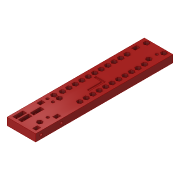
# Autodesk Inventor part: Coupler lift long for bracket right
Saved by Autodesk Inventor 2020 (Build 240168000, 168)
## iProperties
Created: 2019-10-02
Part Number: Coupler lift long for bracket right
Material: Generic
Document SubType Name: Modeling
Designer: ball
Density: 1 g/cm^3
Appearance: Default
Author: ball
Autodesk Inventor part; units mm, degrees
ref_plane "YZ Plane" through (0, 0, 0) normal (1, 0, 0) x (0, 1, 0)
ref_plane "XZ Plane" through (0, 0, 0) normal (0, 1, 0) x (-1, 0, 0)
ref_plane "XY Plane" through (0, 0, 0) normal (0, 0, 1) x (1, 0, 0)
sketch "Sketch1" plane through (0, 0, 0) normal (0, 1, 0) x (-1, 0, 0)
  line L0 (0, 0) -> (35.5, 0)
  line L1 (35.5, 0) -> (35.5, -170)
  line L2 (35.5, -170) -> (0, -170)
  line L3 (0, -170) -> (0, 0)
  dimension "d0" = 35.5
  dimension "d1" = 170
  constraints: 8 end point, 2 parallel, 1 horizontal, 1 perpendicular
  measures "d0" distance of L1.end L2.end
  measures "d1" distance of L0.end L1.end
extrude "BlockShape" add sketch "Sketch1" along normal blind 9
sketch "Sketch2" plane through (0, 9, 0) normal (0, 1, 0) x (1, 0, 0)
  circle A0 centre (-10, 15) radius 3.25 construction
  line L0 (-35.5, 0) -> (0, 0) projected
  line L1 (0, 0) -> (0, 170) projected
  line L2 (-13.25, 15) -> (-11.625, 17.8146)
  line L3 (-11.625, 17.8146) -> (-8.375, 17.8146)
  line L4 (-8.375, 17.8146) -> (-6.75, 15)
  line L5 (-6.75, 15) -> (-8.375, 12.1854)
  line L6 (-8.375, 12.1854) -> (-11.625, 12.1854)
  line L7 (-11.625, 12.1854) -> (-13.25, 15)
  circle A1 centre (-10, 150) radius 3.25 construction
  line L8 (-13.25, 150) -> (-11.625, 152.8146)
  line L9 (-11.625, 152.8146) -> (-8.375, 152.8146)
  line L10 (-8.375, 152.8146) -> (-6.75, 150)
  line L11 (-6.75, 150) -> (-8.375, 147.1854)
  line L12 (-8.375, 147.1854) -> (-11.625, 147.1854)
  line L13 (-11.625, 147.1854) -> (-13.25, 150)
  line L14 (0, 170) -> (-35.5, 170) projected
  circle A2 centre (-10, 15) radius 1.7 construction
  circle A3 centre (-10, 150) radius 1.7 construction
  dimension "d7" = 6.5
  dimension "d10" = 6.5
  dimension "d23" = 135
  dimension "d24" = 15
  dimension "d25" = 10
  dimension "d28" = 3.4
  dimension "d29" = 3.4
  constraints: 24 end point, 4 coincident, 2 centre point, 2 horizontal alignment, 30 other
  measures "d23" distance of point (-10, 150) point (-10, 15)
  measures "d24" distance from line of L0 point (-10, 15)
  measures "d25" distance from line of L1 point (-10, 15)
  measures "d28" diameter of A2
  measures "d29" diameter of A3
extrude "SlideNutWell2" cut sketch "Sketch2" against normal blind 5
sketch "Sketch3" plane through (0, 0, 0) normal (0, -1, 0) x (1, 0, 0)
  circle A0 centre (-10, -25) radius 3.25 construction
  line L0 (0, 0) -> (-35.5, 0) projected
  line L1 (-35.5, 0) -> (-35.5, -170) projected
  line L2 (-11.6286, -27.8125) -> (-13.25, -24.9958)
  line L3 (-13.25, -24.9958) -> (-11.6214, -22.1833)
  line L4 (-11.6214, -22.1833) -> (-8.3714, -22.1875)
  line L5 (-8.3714, -22.1875) -> (-6.75, -25.0042)
  line L6 (-6.75, -25.0042) -> (-8.3786, -27.8167)
  line L7 (-8.3786, -27.8167) -> (-11.6286, -27.8125)
  circle A1 centre (-10, -160) radius 3.25 construction
  line L8 (-6.75, -160) -> (-8.375, -162.8146)
  line L9 (-8.375, -162.8146) -> (-11.625, -162.8146)
  line L10 (-11.625, -162.8146) -> (-13.25, -160)
  line L11 (-13.25, -160) -> (-11.625, -157.1854)
  line L12 (-11.625, -157.1854) -> (-8.375, -157.1854)
  line L13 (-8.375, -157.1854) -> (-6.75, -160)
  line L14 (0, -170) -> (0, 0) projected
  dimension "d15" = 6.5
  dimension "d18" = 6.5
  dimension "d16" = 25
  dimension "d19" = 135
  dimension "d26" = 10
  dimension "d27" = 10
  constraints: 24 end point, 2 coincident, 1 horizontal alignment, 31 other
  measures "d16" distance from line of L0 point (-10, -25)
  measures "d19" distance of point (-10, -160) point (-10, -25)
  measures "d26" distance from line of L14 point (-10, -25)
  measures "d27" distance from line of L14 point (-10, -160)
extrude "SlideNutWell1" cut sketch "Sketch3" against normal blind 5
sketch "Sketch5" plane through (0, 9, 0) normal (0, 1, 0) x (1, 0, 0)
  circle A0 centre (-10, 15) radius 1.7
  line L0 (0, 0) -> (0, 170) projected
  line L1 (-35.5, 0) -> (0, 0) projected
  circle A1 centre (-10, 150) radius 1.7
  circle A2 centre (-10, 25) radius 1.7
  circle A3 centre (-10, 160) radius 1.7
  dimension "d30" = 3.4
  dimension "d31" = 10
  dimension "d32" = 15
  dimension "d33" = 3.4
  dimension "d34" = 10
  dimension "d35" = 135
  dimension "d36" = 3.4
  dimension "d37" = 25
  dimension "d38" = 3.4
  dimension "d39" = 10
  dimension "d40" = 135
  constraints: 4 centre point
  measures "d30" diameter of A0
  measures "d31" distance from line of L0 A0.centre
  measures "d32" distance from line of L1 A0.centre
  measures "d33" diameter of A1
  measures "d34" distance from line of L0 A1.centre
  measures "d35" distance of A1.centre A0.centre
  measures "d36" diameter of A2
  measures "d37" distance from line of L1 A2.centre
  measures "d38" diameter of A3
  measures "d39" distance from line of L0 A3.centre
  measures "d40" distance of A2.centre A3.centre
extrude "SlideMoutingHoles" cut sketch "Sketch5" against normal through all
sketch "Sketch6" plane through (0, 9, 0) normal (0, 1, 0) x (1, 0, 0)
  line L0 (-32.5, 4) -> (-27.7502, 4)
  line L1 (-27.7502, 4) -> (-27.7502, 16.7)
  line L2 (-27.7502, 16.7) -> (-32.5, 16.7)
  line L3 (-32.5, 16.7) -> (-32.5, 4)
  line L4 (-35.5, 0) -> (0, 0) projected
  line L5 (-35.5, 170) -> (-35.5, 0) projected
  line L6 (-25.7502, 4) -> (-21.0002, 4)
  line L7 (-21.0002, 4) -> (-21.0002, 16.7)
  line L8 (-21.0002, 16.7) -> (-25.7502, 16.7)
  line L9 (-25.7502, 16.7) -> (-25.7502, 4)
  line L10 (0, 0) -> (0, 170) construction
  line L11 (-35.5, 170) -> (0, 170) projected
  line L12 (0, 0) -> (-20, 0) construction
  line L13 (-20, 0) -> (-20, 170) construction
  line L14 (-20, 170) -> (0, 170) construction
  line L15 (0, 170) -> (0, 0)
  circle A0 centre (-23.3752, 44.7) radius 1.7
  circle A1 centre (-30.125, 44.7) radius 1.7
  circle A2 centre (-30.125, 52.7) radius 1.7
  circle A3 centre (-23.3752, 52.7) radius 1.7
  line L16 (-25.7502, 18.7) -> (-21.0002, 18.7)
  line L17 (-21.0002, 18.7) -> (-21.0002, 31.4)
  line L18 (-21.0002, 31.4) -> (-25.7502, 31.4)
  line L19 (-25.7502, 31.4) -> (-25.7502, 18.7)
  dimension "d43" = 4.7498
  dimension "d44" = 12.7
  dimension "d45" = 4
  dimension "d46" = 3
  dimension "d47" = 4.75
  dimension "d48" = 2
  dimension "d49" = 20
  dimension "d50" = 3.4
  dimension "d51" = 28
  dimension "d87" = 3.4
  dimension "d88" = 5.375
  dimension "d90" = 3.4
  dimension "d91" = 8
  dimension "d92" = 3.4
  dimension "d180" = 4.75
  dimension "d181" = 12.7
  dimension "d182" = 2
  dimension "d183" = 12.7
  dimension "d184" = 4
  dimension "d260" = 28
  dimension "d261" = 8
  constraints: 32 end point, 8 parallel, 4 centre point, 4 horizontal, 4 perpendicular, 2 point on line
  measures "d43" distance of L2.end L1.end
  measures "d44" distance of L1.end L0.end
  measures "d45" distance between parallel lines of L4 L0
  measures "d46" distance between parallel lines of L5 L3
  measures "d47" distance of L8.end L7.end
  measures "d48" distance between parallel lines of L9 L1
  measures "d49" distance of L13.end L14.end
  measures "d50" diameter of A0
  measures "d51" distance from line of A0.centre L8
  measures "d87" diameter of A1
  measures "d88" distance from line of L5 A1.centre
  measures "d90" diameter of A2
  measures "d91" distance of A2.centre A1.centre
  measures "d92" diameter of A3
  measures "d180" distance of L18.end L17.end
  measures "d181" distance of L17.end L16.end
  measures "d182" distance between parallel lines of L16 L8
  measures "d183" distance between parallel lines of L8 L6
  measures "d184" distance between parallel lines of L4 L6
  measures "d260" distance from line of L2 A1.centre
  measures "d261" distance of A0.centre A3.centre
extrude "PulleyHoles" cut sketch "Sketch6" against normal through all contours L3 L2 L1 L0 | L9 L8 L7 L6 | A0 | A1 | A2 | A3 | L19 L18 L17 L16
sketch "Sketch7" plane through (0, 0, 0) normal (0, -1, 0) x (1, 0, 0)
  circle A0 centre (-23.3752, -44.7) radius 1.7 projected
  circle A1 centre (-23.3752, -44.7) radius 3.25 construction
  circle A2 centre (-30.1625, -44.7) radius 3.25 construction
  line L0 (-30.125, -41.4502) -> (-27.3294, -43.1076)
  line L1 (-27.3294, -43.1076) -> (-27.3669, -46.3574)
  line L2 (-27.3669, -46.3574) -> (-30.2, -47.9498)
  line L3 (-30.2, -47.9498) -> (-32.9956, -46.2924)
  line L4 (-32.9956, -46.2924) -> (-32.9581, -43.0426)
  line L5 (-32.9581, -43.0426) -> (-30.125, -41.4502)
  circle A3 centre (-30.125, -44.7) radius 1.7 projected
  line L6 (-20.1252, -44.7) -> (-21.7502, -47.5146)
  line L7 (-21.7502, -47.5146) -> (-25.0002, -47.5146)
  line L8 (-25.0002, -47.5146) -> (-26.6252, -44.7)
  line L9 (-26.6252, -44.7) -> (-25.0002, -41.8854)
  line L10 (-25.0002, -41.8854) -> (-21.7502, -41.8854)
  line L11 (-21.7502, -41.8854) -> (-20.1252, -44.7)
  point P0 (0, 0)
  dimension "d54" = 6.5
  dimension "d89" = 6.5
  dimension "d262" = 0
  constraints: 24 end point, 4 coincident, 1 horizontal alignment, 32 other
  measures "d262" vertical distance of point (-30.162, -44.7) A3.centre
extrude "TensionNutWells2" cut sketch "Sketch7" against normal blind 5 contours A0 | L0 L1 L2 L3 L4 L5 | A3 | L6 L7 L8 L9 L10 L11
sketch "Sketch8" plane through (-35.5, 0, -170) normal (-1, 0, 0) x (0, 0, 1)
  circle A0 centre (159.65, 4.5) radius 1.4605
  line L0 (0, 9) -> (170, 9) projected
  line L1 (170, 0) -> (170, 9) projected
  circle A1 centre (144.95, 4.5) radius 1.45
  dimension "d57" = 2.921
  dimension "d58" = 4.5
  dimension "d59" = 10.35
  dimension "d185" = 2.9
  dimension "d186" = 14.7
  dimension "d187" = 4.5
  constraints: 2 centre point
  measures "d57" diameter of A0
  measures "d58" distance from line of L0 A0.centre
  measures "d59" distance from line of L1 A0.centre
  measures "d185" diameter of A1
  measures "d186" distance of A1.centre A0.centre
  measures "d187" distance from line of L0 A1.centre
hole "PulleyMountingHole" at (-35.5, 4.5, -10.35) at (-35.5, 4.5, -25.05) direction (1, 0, 0) diameter 2.921 depth 21 counterbore diameter 3.4 counterbore depth 1.5
sketch "Sketch9" plane through (-21.0002, 9, -16.7) normal (-1, 0, 0) x (0, 0, 1)
  circle A0 centre (6.35, -4.5) radius 1.4605 projected
  circle A1 centre (6.35, -4.5) radius 2.54
  circle A2 centre (-8.35, -4.5) radius 1.4605 projected
  circle A3 centre (-8.35, -4.5) radius 2.54
  point P0 (16.7, -9)
  dimension "d67" = 5.08
  dimension "d194" = 5.08
  constraints: 2 centre point, 2 coincident
  measures "d67" diameter of A1
  measures "d194" diameter of A3
extrude "PulleyStandoff4" add sketch "Sketch9" along normal blind 0.2032
sketch "Sketch11" plane through (-25.7502, 9, -4) normal (1, 0, 0) x (0, 0, -1)
  circle A0 centre (6.35, -4.5) radius 2.54
  circle A1 centre (6.35, -4.5) radius 1.4605
  circle A2 centre (21.05, -4.5) radius 1.4605 projected
  circle A3 centre (21.05, -4.5) radius 2.54
  point P0 (-4, -9)
  dimension "d73" = 5.08
  dimension "d195" = 5.08
  constraints: 3 centre point, 3 coincident
  measures "d73" diameter of A0
  measures "d195" diameter of A3
sketch "Sketch12" plane through (-32.5, 9, -4) normal (1, 0, 0) x (0, 0, -1)
  circle A0 centre (6.35, -4.5) radius 2.54
  circle A1 centre (6.35, -4.5) radius 1.4605
  point P0 (-4, -9)
  dimension "d76" = 5.08
  constraints: 2 centre point, 1 coincident
  measures "d76" diameter of A0
extrude "PulleyStandoff1" add sketch "Sketch12" along normal blind 0.2032
sketch "Sketch10" plane through (-27.7502, 9, -16.7) normal (-1, 0, 0) x (0, 0, 1)
  circle A0 centre (6.35, -4.5) radius 2.54
  circle A1 centre (6.35, -4.5) radius 1.4605
  point P0 (16.7, -9)
  dimension "d70" = 5.08
  constraints: 2 centre point, 2 coincident
  measures "d70" diameter of A0
extrude "PulleyStandoff2" add sketch "Sketch10" along normal blind 0.2032
extrude "PulleyStandoff3" add sketch "Sketch11" along normal blind 0.2032
sketch "Sketch14" plane through (0, 0, -170) normal (0, 0, -1) x (-1, 0, 0)
  circle A0 centre (18, 4.5) radius 2.25
  line L0 (35.5, 0) -> (0, 0) projected
  line L1 (0, 0) -> (0, 9) projected
  dimension "d82" = 4.5
  dimension "d83" = 4.5
  dimension "d84" = 18
  constraints: 1 centre point
  measures "d82" diameter of A0
  measures "d83" distance from line of L0 A0.centre
  measures "d84" distance from line of L1 A0.centre
extrude "4mmShaftHole" cut sketch "Sketch14" against normal blind 71
sketch "Sketch15" plane through (0, 9, 0) normal (0, 1, 0) x (1, 0, 0)
  circle A0 centre (-30.125, 52.7) radius 1.7 projected
  circle A1 centre (-30.125, 52.7) radius 3.25 construction
  circle A2 centre (-23.3752, 52.7) radius 1.7 projected
  circle A3 centre (-23.3752, 52.7) radius 3.25 construction
  line L0 (-30.125, 49.45) -> (-32.9396, 51.075)
  line L1 (-32.9396, 51.075) -> (-32.9396, 54.325)
  line L2 (-32.9396, 54.325) -> (-30.125, 55.95)
  line L3 (-30.125, 55.95) -> (-27.3104, 54.325)
  line L4 (-27.3104, 54.325) -> (-27.3104, 51.075)
  line L5 (-27.3104, 51.075) -> (-30.125, 49.45)
  line L6 (-23.3752, 49.45) -> (-26.1898, 51.075)
  line L7 (-26.1898, 51.075) -> (-26.1898, 54.325)
  line L8 (-26.1898, 54.325) -> (-23.3752, 55.95)
  line L9 (-23.3752, 55.95) -> (-20.5606, 54.325)
  line L10 (-20.5606, 54.325) -> (-20.5606, 51.075)
  line L11 (-20.5606, 51.075) -> (-23.3752, 49.45)
  point P0 (0, 0)
  dimension "d93" = 6.5
  dimension "d94" = 6.5
  constraints: 24 end point, 4 coincident, 2 vertical alignment, 30 other
extrude "TensionNutWells1" cut sketch "Sketch15" against normal blind 5
ref_plane "PulleyMidPlane1" through (-30.1251, 9, -4) normal (1, 0, 0) x (0, 0, -1)
ref_plane "PulleyMidPlane2" through (-23.3752, 9, -16.7) normal (-1, 0, 0) x (0, 0, 1)
ref_plane "Work Plane3" through (-7.7, 0, 0) normal (1, 0, 0) x (0, 0, -1)
sketch "Sketch20" plane through (-7.7, 0, 0) normal (1, 0, 0) x (0, 0, -1)
  circle A0 centre (6.65, 4.5) radius 3.45 construction
  line L0 (0, 0) -> (0, 9) construction
  line L1 (0, 0) -> (170, 0) construction
  line L2 (6.65, 1.05) -> (3.6622, 2.775)
  line L3 (3.6622, 2.775) -> (3.6622, 9)
  line L4 (9.6378, 9) -> (9.6378, 2.775)
  line L5 (9.6378, 2.775) -> (6.65, 1.05)
  line L6 (170, 9) -> (0, 9) projected
  line L7 (3.6622, 9) -> (9.6378, 9)
  line L8 (147.1854, 9) -> (147.1854, 4) construction
  circle A1 centre (31.6858, 4.5) radius 3.45 construction
  circle A2 centre (31.6858, 4.5) radius 3.45 construction
  line L9 (31.6858, 1.05) -> (28.698, 2.775)
  line L10 (28.698, 2.775) -> (28.698, 9)
  line L11 (34.6736, 9) -> (34.6736, 2.775)
  line L12 (34.6736, 2.775) -> (31.6858, 1.05)
  line L13 (28.698, 9) -> (34.6736, 9)
  dimension "d199" = 6.9
  dimension "d279" = 6.9
  dimension "d200" = 6.65
  dimension "d201" = 4.5
  dimension "d276" = 6.9
  dimension "d277" = 31.6858
  dimension "d278" = 4.5
  constraints: 20 end point, 2 coincident, 2 point on line, 2 vertical alignment, 1 centre point, 16 other
  measures "d200" distance from line of L0 point (6.65, 4.5)
  measures "d201" distance from line of L1 point (6.65, 4.5)
  measures "d276" diameter of A1
  measures "d277" distance from line of L0 A1.centre
  measures "d278" distance from line of L1 A1.centre
extrude "NutWellsNonPulleySide" cut sketch "Sketch20" along normal blind 4.4
sketch "Sketch21" plane through (0, 0, 0) normal (1, 0, 0) x (0, 0, -1)
  line L0 (3.6622, 9) -> (3.6622, 2.775) construction
  line L1 (9.6378, 2.775) -> (9.6378, 9) construction
  circle A0 centre (6.65, 4.5) radius 1.7
  line L2 (170, 0) -> (0, 0) projected
  line L3 (27.8167, 0) -> (27.8167, 5) construction
  circle A1 centre (31.6858, 4.5) radius 1.7
  line L4 (0, 0) -> (0, 9) projected
  dimension "d210" = 3.4
  dimension "d211" = 5.9756
  dimension "d212" = 2.9878
  dimension "d213" = 4.5
  dimension "d272" = 3.4
  dimension "d274" = 4.5
  dimension "d275" = 31.6858
  constraints: 2 centre point
  measures "d210" diameter of A0
  measures "d211" distance between parallel lines of L1 L0
  measures "d212" distance from line of L0 A0.centre
  measures "d213" distance from line of L2 A0.centre
  measures "d272" diameter of A1
  measures "d274" distance from line of L2 A1.centre
  measures "d275" distance from line of L4 A1.centre
extrude "NutWellHolesNonPulleySide" cut sketch "Sketch21" against normal blind 8.4
ref_plane "Work Plane4" through (-27.8, 0, -170) normal (-1, 0, 0) x (0, 0, 1)
sketch "Sketch22" plane through (-35.5, 0, -170) normal (-1, 0, 0) x (0, 0, 1)
  line L0 (170, 0) -> (0, 0) projected
  line L1 (0, 9) -> (170, 9) projected
  line L2 (0, 0) -> (0, 9) projected
  line L3 (138.6, 9) -> (138.6, 0) construction
  line L4 (128.5498, 0) -> (128.5498, 5) construction
  circle A0 centre (133.5749, 4.5) radius 1.7
  circle A1 centre (16, 4.5) radius 1.7
  dimension "d225" = 9
  dimension "d263" = 3.4
  dimension "d264" = 4.5
  dimension "d265" = 10.0502
  dimension "d266" = 5.0251
  dimension "d306" = 3.4
  dimension "d307" = 16
  dimension "d308" = 4.5
  constraints: 2 centre point
  measures "d225" distance between parallel lines of L0 L1
  measures "d263" diameter of A0
  measures "d264" distance from line of L0 A0.centre
  measures "d265" distance between parallel lines of L3 L4
  measures "d266" distance from line of L4 A0.centre
  measures "d306" diameter of A1
  measures "d307" distance from line of L2 A1.centre
  measures "d308" distance from line of L0 A1.centre
extrude "NutWellHolesPulleySide" cut sketch "Sketch22" against normal blind 8.4
sketch "Sketch23" plane through (-27.8, 0, -170) normal (-1, 0, 0) x (0, 0, 1)
  line L0 (170, 9) -> (0, 9) projected
  circle A0 centre (133.5749, 4.5) radius 1.7 construction
  circle A1 centre (133.5749, 4.5) radius 3.45 construction
  line L1 (133.5749, 1.05) -> (130.5871, 2.775)
  line L2 (130.5871, 2.775) -> (130.5871, 9)
  line L3 (136.5627, 9) -> (136.5627, 2.775)
  line L4 (136.5627, 2.775) -> (133.5749, 1.05)
  line L5 (130.5871, 9) -> (136.5627, 9)
  circle A2 centre (16, 4.5) radius 1.7 construction
  line L6 (13.0122, 2.775) -> (13.0122, 9)
  line L7 (16, 1.05) -> (13.0122, 2.775)
  circle A3 centre (16, 4.5) radius 3.45 construction
  line L8 (13.0122, 9) -> (18.9878, 9)
  line L9 (18.9878, 9) -> (18.9878, 2.775)
  line L10 (18.9878, 2.775) -> (16, 1.05)
  point P0 (170, 0)
  constraints: 20 end point, 4 coincident, 2 vertical alignment, 4 other
extrude "NutWellsPulleySide" cut sketch "Sketch23" along normal blind 4.4
sketch "Sketch25" plane through (0, 9, 0) normal (0, 1, 0) x (1, 0, 0)
  circle A0 centre (-28.5, 61.7) radius 1.7
  circle A1 centre (-23.3752, 52.7) radius 1.7 projected
  line L0 (-35.5, 170) -> (-35.5, 0) projected
  circle A2 centre (-7, 61.7) radius 1.7
  line L1 (0, 0) -> (0, 170) projected
  circle A3 centre (-28.5, 69.7) radius 1.7
  circle A4 centre (-7, 69.7) radius 1.7
  circle A5 centre (-28.5, 77.7) radius 1.7
  circle A6 centre (-7, 77.7) radius 1.7
  circle A7 centre (-28.5, 85.7) radius 1.7
  circle A8 centre (-7, 85.7) radius 1.7
  circle A9 centre (-28.5, 93.7) radius 1.7
  circle A10 centre (-7, 93.7) radius 1.7
  circle A11 centre (-28.5, 101.7) radius 1.7
  circle A12 centre (-7, 101.7) radius 1.7
  circle A13 centre (-28.5, 109.7) radius 1.7
  circle A14 centre (-7, 109.7) radius 1.7
  circle A15 centre (-28.5, 117.7) radius 1.7
  circle A16 centre (-7, 117.7) radius 1.7
  circle A17 centre (-28.5, 125.7) radius 1.7
  circle A18 centre (-7, 125.7) radius 1.7
  circle A19 centre (-28.5, 133.7) radius 1.7
  circle A20 centre (-7, 133.7) radius 1.7
  circle A21 centre (-28.5, 141.7) radius 1.7
  circle A22 centre (-7, 141.7) radius 1.7
  circle A23 centre (-28.5, 149.7) radius 1.7
  circle A24 centre (-7, 149.7) radius 1.7
  circle A25 centre (-28.5, 157.7) radius 1.7
  circle A26 centre (-7, 157.7) radius 1.7
  circle A27 centre (-28.5, 165.7) radius 1.7
  circle A28 centre (-7, 165.7) radius 1.7
  dimension "d280" = 3.4
  dimension "d281" = 9
  dimension "d282" = 7
  dimension "d283" = 3.4
  dimension "d284" = 9
  dimension "d285" = 7
  dimension "d288" = 8
  constraints: 28 centre point, 1 vertical, 52 other
  measures "d280" diameter of A0
  measures "d281" vertical distance of A1.centre A0.centre
  measures "d282" distance from line of L0 A0.centre
  measures "d283" diameter of A2
  measures "d284" vertical distance of A2.centre A1.centre
  measures "d285" distance from line of L1 A2.centre
  measures "d288" distance of A0.centre A3.centre
extrude "BracketMountingHoles" cut sketch "Sketch25" against normal through all contours A0 | A2 | A3 | A4 | A5 | A6 | A7 | A8 | A9 | A10 | A11 | A12 | A13 | A14 | A15 | A16 | A17 | A18 | A19 | A20 | A21 | A22 | A27 | A28
sketch "Sketch26" plane through (0, 9, 0) normal (0, 1, 0) x (1, 0, 0)
  circle A0 centre (-28.5, 61.7) radius 1.7 construction
  circle A1 centre (-7, 61.7) radius 1.7 construction
  circle A2 centre (-28.5, 61.7) radius 3.25 construction
  circle A3 centre (-7, 61.7) radius 3.25 construction
  line L0 (-28.5, 64.95) -> (-25.6854, 63.325)
  line L1 (-25.6854, 63.325) -> (-25.6854, 60.075)
  line L2 (-25.6854, 60.075) -> (-28.5, 58.45)
  line L3 (-28.5, 58.45) -> (-31.3146, 60.075)
  line L4 (-31.3146, 60.075) -> (-31.3146, 63.325)
  line L5 (-31.3146, 63.325) -> (-28.5, 64.95)
  circle A4 centre (-7, 61.7) radius 1.7 projected
  line L6 (-7, 64.95) -> (-4.1854, 63.325)
  line L7 (-4.1854, 63.325) -> (-4.1854, 60.075)
  line L8 (-4.1854, 60.075) -> (-7, 58.45)
  line L9 (-7, 58.45) -> (-9.8146, 60.075)
  line L10 (-9.8146, 60.075) -> (-9.8146, 63.325)
  line L11 (-9.8146, 63.325) -> (-7, 64.95)
  line L12 (0, 0) -> (0, 170) construction
  line L13 (-4.1854, 71.325) -> (-4.1854, 68.075)
  line L14 (-4.1854, 68.075) -> (-7, 66.45)
  line L15 (-7, 66.45) -> (-9.8146, 68.075)
  line L16 (-9.8146, 68.075) -> (-9.8146, 71.325)
  line L17 (-9.8146, 71.325) -> (-7, 72.95)
  line L18 (-7, 72.95) -> (-4.1854, 71.325)
  line L19 (-31.3146, 68.075) -> (-31.3146, 71.325)
  line L20 (-28.5, 66.45) -> (-31.3146, 68.075)
  line L21 (-31.3146, 71.325) -> (-28.5, 72.95)
  line L22 (-28.5, 72.95) -> (-25.6854, 71.325)
  line L23 (-25.6854, 68.075) -> (-28.5, 66.45)
  line L24 (-25.6854, 71.325) -> (-25.6854, 68.075)
  line L25 (-4.1854, 79.325) -> (-4.1854, 76.075)
  line L26 (-4.1854, 76.075) -> (-7, 74.45)
  line L27 (-7, 74.45) -> (-9.8146, 76.075)
  line L28 (-9.8146, 76.075) -> (-9.8146, 79.325)
  line L29 (-9.8146, 79.325) -> (-7, 80.95)
  line L30 (-7, 80.95) -> (-4.1854, 79.325)
  line L31 (-31.3146, 76.075) -> (-31.3146, 79.325)
  line L32 (-28.5, 74.45) -> (-31.3146, 76.075)
  line L33 (-31.3146, 79.325) -> (-28.5, 80.95)
  line L34 (-28.5, 80.95) -> (-25.6854, 79.325)
  line L35 (-25.6854, 76.075) -> (-28.5, 74.45)
  line L36 (-25.6854, 79.325) -> (-25.6854, 76.075)
  line L37 (-4.1854, 87.325) -> (-4.1854, 84.075)
  line L38 (-4.1854, 84.075) -> (-7, 82.45)
  line L39 (-7, 82.45) -> (-9.8146, 84.075)
  line L40 (-9.8146, 84.075) -> (-9.8146, 87.325)
  line L41 (-9.8146, 87.325) -> (-7, 88.95)
  line L42 (-7, 88.95) -> (-4.1854, 87.325)
  line L43 (-31.3146, 84.075) -> (-31.3146, 87.325)
  line L44 (-28.5, 82.45) -> (-31.3146, 84.075)
  line L45 (-31.3146, 87.325) -> (-28.5, 88.95)
  line L46 (-28.5, 88.95) -> (-25.6854, 87.325)
  line L47 (-25.6854, 84.075) -> (-28.5, 82.45)
  line L48 (-25.6854, 87.325) -> (-25.6854, 84.075)
  line L49 (-4.1854, 95.325) -> (-4.1854, 92.075)
  line L50 (-4.1854, 92.075) -> (-7, 90.45)
  line L51 (-7, 90.45) -> (-9.8146, 92.075)
  line L52 (-9.8146, 92.075) -> (-9.8146, 95.325)
  line L53 (-9.8146, 95.325) -> (-7, 96.95)
  line L54 (-7, 96.95) -> (-4.1854, 95.325)
  line L55 (-31.3146, 92.075) -> (-31.3146, 95.325)
  line L56 (-28.5, 90.45) -> (-31.3146, 92.075)
  line L57 (-31.3146, 95.325) -> (-28.5, 96.95)
  line L58 (-28.5, 96.95) -> (-25.6854, 95.325)
  line L59 (-25.6854, 92.075) -> (-28.5, 90.45)
  line L60 (-25.6854, 95.325) -> (-25.6854, 92.075)
  line L61 (-4.1854, 103.325) -> (-4.1854, 100.075)
  line L62 (-4.1854, 100.075) -> (-7, 98.45)
  line L63 (-7, 98.45) -> (-9.8146, 100.075)
  line L64 (-9.8146, 100.075) -> (-9.8146, 103.325)
  line L65 (-9.8146, 103.325) -> (-7, 104.95)
  line L66 (-7, 104.95) -> (-4.1854, 103.325)
  line L67 (-31.3146, 100.075) -> (-31.3146, 103.325)
  line L68 (-28.5, 98.45) -> (-31.3146, 100.075)
  line L69 (-31.3146, 103.325) -> (-28.5, 104.95)
  line L70 (-28.5, 104.95) -> (-25.6854, 103.325)
  line L71 (-25.6854, 100.075) -> (-28.5, 98.45)
  line L72 (-25.6854, 103.325) -> (-25.6854, 100.075)
  line L73 (-4.1854, 111.325) -> (-4.1854, 108.075)
  line L74 (-4.1854, 108.075) -> (-7, 106.45)
  line L75 (-7, 106.45) -> (-9.8146, 108.075)
  line L76 (-9.8146, 108.075) -> (-9.8146, 111.325)
  line L77 (-9.8146, 111.325) -> (-7, 112.95)
  line L78 (-7, 112.95) -> (-4.1854, 111.325)
  line L79 (-31.3146, 108.075) -> (-31.3146, 111.325)
  line L80 (-28.5, 106.45) -> (-31.3146, 108.075)
  line L81 (-31.3146, 111.325) -> (-28.5, 112.95)
  line L82 (-28.5, 112.95) -> (-25.6854, 111.325)
  line L83 (-25.6854, 108.075) -> (-28.5, 106.45)
  line L84 (-25.6854, 111.325) -> (-25.6854, 108.075)
  line L85 (-4.1854, 119.325) -> (-4.1854, 116.075)
  line L86 (-4.1854, 116.075) -> (-7, 114.45)
  line L87 (-7, 114.45) -> (-9.8146, 116.075)
  line L88 (-9.8146, 116.075) -> (-9.8146, 119.325)
  line L89 (-9.8146, 119.325) -> (-7, 120.95)
  line L90 (-7, 120.95) -> (-4.1854, 119.325)
  line L91 (-31.3146, 116.075) -> (-31.3146, 119.325)
  line L92 (-28.5, 114.45) -> (-31.3146, 116.075)
  line L93 (-31.3146, 119.325) -> (-28.5, 120.95)
  line L94 (-28.5, 120.95) -> (-25.6854, 119.325)
  line L95 (-25.6854, 116.075) -> (-28.5, 114.45)
  line L96 (-25.6854, 119.325) -> (-25.6854, 116.075)
  line L97 (-4.1854, 127.325) -> (-4.1854, 124.075)
  line L98 (-4.1854, 124.075) -> (-7, 122.45)
  line L99 (-7, 122.45) -> (-9.8146, 124.075)
  line L100 (-9.8146, 124.075) -> (-9.8146, 127.325)
  line L101 (-9.8146, 127.325) -> (-7, 128.95)
  line L102 (-7, 128.95) -> (-4.1854, 127.325)
  line L103 (-31.3146, 124.075) -> (-31.3146, 127.325)
  line L104 (-28.5, 122.45) -> (-31.3146, 124.075)
  line L105 (-31.3146, 127.325) -> (-28.5, 128.95)
  line L106 (-28.5, 128.95) -> (-25.6854, 127.325)
  line L107 (-25.6854, 124.075) -> (-28.5, 122.45)
  line L108 (-25.6854, 127.325) -> (-25.6854, 124.075)
  line L109 (-4.1854, 135.325) -> (-4.1854, 132.075)
  line L110 (-4.1854, 132.075) -> (-7, 130.45)
  line L111 (-7, 130.45) -> (-9.8146, 132.075)
  line L112 (-9.8146, 132.075) -> (-9.8146, 135.325)
  line L113 (-9.8146, 135.325) -> (-7, 136.95)
  line L114 (-7, 136.95) -> (-4.1854, 135.325)
  line L115 (-31.3146, 132.075) -> (-31.3146, 135.325)
  line L116 (-28.5, 130.45) -> (-31.3146, 132.075)
  line L117 (-31.3146, 135.325) -> (-28.5, 136.95)
  line L118 (-28.5, 136.95) -> (-25.6854, 135.325)
  line L119 (-25.6854, 132.075) -> (-28.5, 130.45)
  line L120 (-25.6854, 135.325) -> (-25.6854, 132.075)
  line L121 (-4.1854, 143.325) -> (-4.1854, 140.075)
  line L122 (-4.1854, 140.075) -> (-7, 138.45)
  line L123 (-7, 138.45) -> (-9.8146, 140.075)
  line L124 (-9.8146, 140.075) -> (-9.8146, 143.325)
  line L125 (-9.8146, 143.325) -> (-7, 144.95)
  line L126 (-7, 144.95) -> (-4.1854, 143.325)
  line L127 (-31.3146, 140.075) -> (-31.3146, 143.325)
  line L128 (-28.5, 138.45) -> (-31.3146, 140.075)
  line L129 (-31.3146, 143.325) -> (-28.5, 144.95)
  line L130 (-28.5, 144.95) -> (-25.6854, 143.325)
  line L131 (-25.6854, 140.075) -> (-28.5, 138.45)
  line L132 (-25.6854, 143.325) -> (-25.6854, 140.075)
  line L133 (-4.1854, 151.325) -> (-4.1854, 148.075)
  line L134 (-4.1854, 148.075) -> (-7, 146.45)
  line L135 (-7, 146.45) -> (-9.8146, 148.075)
  line L136 (-9.8146, 148.075) -> (-9.8146, 151.325)
  line L137 (-9.8146, 151.325) -> (-7, 152.95)
  line L138 (-7, 152.95) -> (-4.1854, 151.325)
  line L139 (-31.3146, 148.075) -> (-31.3146, 151.325)
  line L140 (-28.5, 146.45) -> (-31.3146, 148.075)
  line L141 (-31.3146, 151.325) -> (-28.5, 152.95)
  line L142 (-28.5, 152.95) -> (-25.6854, 151.325)
  line L143 (-25.6854, 148.075) -> (-28.5, 146.45)
  line L144 (-25.6854, 151.325) -> (-25.6854, 148.075)
  line L145 (-4.1854, 159.325) -> (-4.1854, 156.075)
  line L146 (-4.1854, 156.075) -> (-7, 154.45)
  line L147 (-7, 154.45) -> (-9.8146, 156.075)
  line L148 (-9.8146, 156.075) -> (-9.8146, 159.325)
  line L149 (-9.8146, 159.325) -> (-7, 160.95)
  line L150 (-7, 160.95) -> (-4.1854, 159.325)
  line L151 (-31.3146, 156.075) -> (-31.3146, 159.325)
  line L152 (-28.5, 154.45) -> (-31.3146, 156.075)
  line L153 (-31.3146, 159.325) -> (-28.5, 160.95)
  line L154 (-28.5, 160.95) -> (-25.6854, 159.325)
  line L155 (-25.6854, 156.075) -> (-28.5, 154.45)
  line L156 (-25.6854, 159.325) -> (-25.6854, 156.075)
  line L157 (-4.1854, 167.325) -> (-4.1854, 164.075)
  line L158 (-4.1854, 164.075) -> (-7, 162.45)
  line L159 (-7, 162.45) -> (-9.8146, 164.075)
  line L160 (-9.8146, 164.075) -> (-9.8146, 167.325)
  line L161 (-9.8146, 167.325) -> (-7, 168.95)
  line L162 (-7, 168.95) -> (-4.1854, 167.325)
  line L163 (-31.3146, 164.075) -> (-31.3146, 167.325)
  line L164 (-28.5, 162.45) -> (-31.3146, 164.075)
  line L165 (-31.3146, 167.325) -> (-28.5, 168.95)
  line L166 (-28.5, 168.95) -> (-25.6854, 167.325)
  line L167 (-25.6854, 164.075) -> (-28.5, 162.45)
  line L168 (-25.6854, 167.325) -> (-25.6854, 164.075)
  dimension "d295" = 6.5
  dimension "d296" = 6.5
  dimension "d299" = 8
  constraints: 336 end point, 4 coincident, 2 vertical alignment, 1 vertical, 342 other
  measures "d299" distance of L6.end L13.start
extrude "BracketNutWells" cut sketch "Sketch26" against normal blind 5 contours L0 L1 L2 L3 L4 L5 | A4 | L6 L7 L8 L9 L10 L11 | L13 L14 L15 L16 L17 L18 | L19 L21 L22 L24 L23 L20 | L25 L26 L27 L28 L29 L30 | L31 L33 L34 L36 L35 L32 | L37 L38 L39 L40 L41 L42 | L43 L45 L46 L48 L47 L44 | L49 L50 L51 L52 L53 L54 | L55 L57 L58 L60 L59 L56 | L61 L62 L63 L64 L65 L66 | L67 L69 L70 L72 L71 L68 | L73 L74 L75 L76 L77 L78 | L79 L81 L82 L84 L83 L80 | L85 L86 L87 L88 L89 L90 | L91 L93 L94 L96 L95 L92 | L97 L98 L99 L100 L101 L102 | L103 L105 L106 L108 L107 L104 | L109 L110 L111 L112 L113 L114 | L115 L117 L118 L120 L119 L116 | L121 L122 L123 L124 L125 L126 | L127 L129 L130 L132 L131 L128 | L157 L158 L159 L160 L161 L162 | L163 L165 L166 L168 L167 L164
sketch "Sketch27" plane through (0, 9, 0) normal (0, 1, 0) x (1, 0, 0)
  line L0 (-10.7111, 88.9618) -> (-23.8474, 88.9618) construction
  line L1 (-23.8474, 88.9618) -> (-23.8474, 88.649) construction
  line L2 (-23.8474, 88.649) -> (-10.7111, 88.649) construction
  line L3 (-10.7111, 88.649) -> (-10.7111, 88.9618) construction
  line L4 (-24.054, 98.8054) -> (-12.4656, 98.8054)
  line L5 (-12.4656, 98.8054) -> (-12.4656, 78.8054)
  line L6 (-12.4656, 78.8054) -> (-15.1237, 78.8054)
  line L7 (-15.1237, 78.8054) -> (-15.1237, 96.4391)
  line L8 (-15.1237, 96.4391) -> (-24.054, 96.4391)
  line L9 (-24.054, 96.4391) -> (-24.054, 98.8054)
  point P0 (0, 0)
  constraints: 2 other
emboss "Emboss1" sketch "Sketch27" operation cut depth 1 direction (0, -1, 0)
equation "\"d183\" = d44"
equation "\"d184\" = d45"
equation "\"d260\" = d51"
equation "\"d261\" = d91"
equation "\"d187\" = d58"
equation "\"d277\" = d275"
equation "\"d278\" = d201"
equation "\"d212\" = 0.5 * d211"
equation "\"d274\" = d213"
equation "\"d264\" = d228"
equation "\"d266\" = 0.5 * d265"
equation "\"d284\" = d281"
equation "\"d285\" = d282"
equation "\"d228\" = 0.5 * d225"
body "Solid1"
